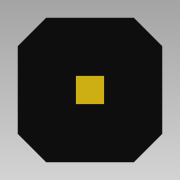
# Autodesk Inventor part: Pin-round-2.54-male
Saved by Autodesk Inventor 2016 (Build 200138000, 138)
## iProperties
Created: 2016-05-26
Part Number: Pin-round-2.54-male
Material: Generic
Document SubType Name: Modeling
Designer: admin
Density: 1 g/cm^3
Appearance: Default
Mass: 0.0173311 g
Surface Area: 0.524462 cm^2
Volume: 0.0173311 cm^3
Author: admin
Autodesk Inventor part; units mm, degrees
ref_plane "YZ Plane" through (0, 0, 0) normal (1, 0, 0) x (0, 1, 0)
ref_plane "XZ Plane" through (0, 0, 0) normal (0, 1, 0) x (-1, 0, 0)
ref_plane "XY Plane" through (0, 0, 0) normal (0, 0, 1) x (1, 0, 0)
sketch "Sketch3" plane through (0, 0, 0) normal (0, 1, 0) x (-1, 0, 0)
  line L0 (0.77, 1.27) -> (-0.77, 1.27)
  line L1 (-1.27, 0.77) -> (-1.27, -0.77)
  line L2 (-0.77, -1.27) -> (0.77, -1.27)
  line L3 (1.27, -0.77) -> (1.27, 0.77)
  line L4 (1.27, 0.77) -> (0.77, 1.27)
  line L5 (-0.77, 1.27) -> (-1.27, 0.77)
  line L6 (-1.27, -0.77) -> (-0.77, -1.27)
  line L7 (0.77, -1.27) -> (1.27, -0.77)
  point P0 (0, 0)
  point P1 (-1.27, 0)
  point P2 (0, -1.27)
  dimension "d6" = 2.54
  dimension "d7" = 0.5
  dimension "d8" = 45
  constraints: 16 end point, 6 perpendicular, 4 parallel, 2 midpoint, 1 horizontal, 1 horizontal alignment, 1 vertical alignment
  measures "d6" distance between parallel lines of L1 L3
  measures "d7" distance from line of L2.end L3
  measures "d8" angle of L4 L3
extrude "Extrusion3" add sketch "Sketch3" along normal blind 2.54
sketch "Sketch4" plane through (0, 2.54, 0) normal (0, 1, 0) x (1, 0, 0)
  line L0 (-0.25, -0.25) -> (0.25, -0.25)
  line L1 (0.25, -0.25) -> (0.25, 0.25)
  line L2 (0.25, 0.25) -> (-0.25, 0.25)
  line L3 (-0.25, 0.25) -> (-0.25, -0.25)
  point P0 (0, 0)
  point P1 (0, 0.25)
  point P2 (-0.25, 0)
  dimension "d11" = 0.5
  constraints: 8 end point, 2 midpoint, 2 parallel, 2 perpendicular, 1 horizontal, 1 horizontal alignment, 1 vertical alignment
  measures "d11" distance of L0.start L0.end
extrude "Extrusion4" add sketch "Sketch4" along normal blind 6.5
sketch "Sketch5" plane through (0, 0, 0) normal (0, -1, 0) x (1, 0, 0)
  circle A0 centre (0, 0) radius 0.25
  dimension "d14" = 0.5
  constraints: 1 centre point, 1 coincident
  measures "d14" diameter of A0
extrude "Extrusion5" add sketch "Sketch5" along normal blind 3
body "Solid2"
